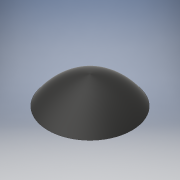
# Autodesk Inventor part: bolt cover
Saved by Autodesk Inventor 2019 (Build 230136000, 136)
## iProperties
Created: 2019-10-24
Part Number: bolt cover
Material: UHMW, Black
Document SubType Name: Modeling
Designer: robgr
Mass: 0.0258386 g
Surface Area: 0.662281 cm^2
Volume: 0.0274879 cm^3
Density: 0.94 g/cm^3
Appearance: Smooth - Black
Author: robgr
Autodesk Inventor part; units mm, degrees
ref_plane "YZ Plane" through (0, 0, 0) normal (1, 0, 0) x (0, 1, 0)
ref_plane "XZ Plane" through (0, 0, 0) normal (0, 1, 0) x (-1, 0, 0)
ref_plane "XY Plane" through (0, 0, 0) normal (0, 0, 1) x (1, 0, 0)
sketch "Sketch1" plane through (0, 0, 0) normal (0, 0, 1) x (1, 0, 0)
  line L0 (0, 0) -> (-3, 0)
  line L1 (-3, 0) -> (-3, 2)
  arc A0 (0, 0) -> (-3, 2) centre (-3.91, -2.615) ccw
  dimension "d0" = 3
  dimension "d1" = 2
  constraints: 4 end point, 2 point on circle, 1 centre point, 1 horizontal, 1 perpendicular
  measures "d0" distance of L0.start L0.end
  measures "d1" distance of L0.end L1.end
revolve "Revolution1" add sketch "Sketch1" angle 360 about axis through (-3, 0, 0) along (0, 1, 0)
body "Solid1"
